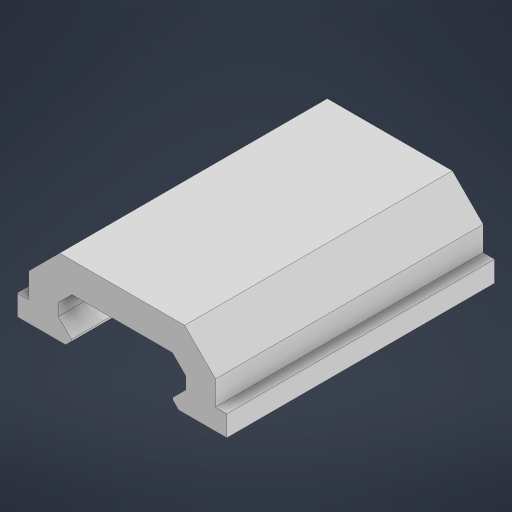
# Autodesk Inventor part: Rail clamp
Saved by Autodesk Inventor 2023 (Build 270158000, 158)
## iProperties
Created: 2023-10-16
Part Number: Rail clamp
Material: Generic
Document SubType Name: Modeling
Designer: nick_
Density: 1 g/cm^3
Appearance: Default
Author: nick_
Autodesk Inventor part; units mm, degrees
ref_plane "YZ Plane" through (0, 0, 0) normal (1, 0, 0) x (0, 1, 0)
ref_plane "XZ Plane" through (0, 0, 0) normal (0, 1, 0) x (-1, 0, 0)
ref_plane "XY Plane" through (0, 0, 0) normal (0, 0, 1) x (1, 0, 0)
sketch "Sketch1" plane through (0, 0, 0) normal (0, 0, 1) x (1, 0, 0)
  line L0 (6.25, -6.1609) -> (-18.75, -6.1609) construction
  line L1 (6.25, -3.1609) -> (6.25, -6.1609) construction
  line L2 (2.1447, -3.1609) -> (6.25, -3.1609) construction
  line L3 (2.1447, -0.2145) -> (2.1447, -3.1609) construction
  line L4 (4.3545, 1.9953) -> (2.1447, -0.2145) construction
  line L5 (4.3545, 3.9511) -> (4.3545, 1.9953) construction
  line L6 (2.1447, 6.1609) -> (4.3545, 3.9511) construction
  line L7 (2.1447, 6.1609) -> (-14.6447, 6.1609) construction
  line L8 (-14.6447, 6.1609) -> (-16.8545, 3.9511) construction
  line L9 (-16.8545, 3.9511) -> (-16.8545, 1.9953) construction
  line L10 (-16.8545, 1.9953) -> (-14.6447, -0.2145) construction
  line L11 (-14.6447, -0.2145) -> (-14.6447, -3.1609) construction
  line L12 (-14.6447, -3.1609) -> (-18.75, -3.1609) construction
  line L13 (-18.75, -3.1609) -> (-18.75, -6.1609) construction
  line L14 (2.2447, -3.0609) -> (6.35, -3.0609)
  line L15 (6.35, -3.0609) -> (6.35, -6.2609)
  line L16 (6.35, -6.2609) -> (-18.85, -6.2609)
  line L17 (-18.85, -6.2609) -> (-18.85, -3.0609)
  line L18 (-18.85, -3.0609) -> (-14.7447, -3.0609)
  line L19 (-14.7447, -3.0609) -> (-14.7447, -0.2559)
  line L20 (-14.7447, -0.2559) -> (-16.9545, 1.9539)
  line L21 (-16.9545, 1.9539) -> (-16.9545, 3.9925)
  line L22 (-16.9545, 3.9925) -> (-14.6861, 6.2609)
  line L23 (-14.6861, 6.2609) -> (2.1861, 6.2609)
  line L24 (2.1861, 6.2609) -> (4.4545, 3.9925)
  line L25 (4.4545, 3.9925) -> (4.4545, 1.9539)
  line L26 (4.4545, 1.9539) -> (2.2447, -0.2559)
  line L27 (2.2447, -0.2559) -> (2.2447, -3.0609)
  line L28 (11.35, 1.9391) -> (9.4545, 1.9391)
  line L29 (9.4545, 1.9391) -> (9.4545, 6.0636)
  line L30 (9.4545, 6.0636) -> (4.2572, 11.2609)
  line L31 (4.2572, 11.2609) -> (-16.7572, 11.2609)
  line L32 (-16.7572, 11.2609) -> (-21.9545, 6.0636)
  line L33 (-21.9545, 6.0636) -> (-21.9545, 1.9391)
  line L34 (-21.9545, 1.9391) -> (-23.85, 1.9391)
  line L35 (-23.85, 1.9391) -> (-23.85, -1.5609)
  line L36 (11.35, -1.5609) -> (11.35, 1.9391)
  line L37 (2.2447, -1.5609) -> (11.35, -1.5609)
  line L38 (-14.7447, -1.5609) -> (-23.85, -1.5609)
  point P0 (0, 0)
  point P1 (6.7974, -1.5609)
  point P2 (-19.2974, -1.5609)
  dimension "d0" = 0.1
  dimension "d1" = 5
  dimension "d2" = 1.5
  dimension "d3" = 5
  dimension "d5" = 5
  constraints: 50 end point, 2 midpoint, 2 perpendicular, 2 point on line, 1 horizontal alignment, 19 other
  measures "d0" distance between parallel lines of L3 L27
  measures "d1" distance between parallel lines of L36 L15
  measures "d2" distance between parallel lines of L37 L14
  measures "d3" distance between parallel lines of L31 L23
  measures "d5" distance between parallel lines of L35 L17
extrude "Extrusion1" add sketch "Sketch1" against normal blind 45 contours L27 L26 L25 L24 L23 L22 L21 L20 L19 L38 L35 L34 L33 L32 L31 L30 L29 L28 L36 L37
chamfer "Chamfer1" distance 1 angle 45 2 edges at (-14.7447, -1.5609, -22.5) (2.2447, -1.5609, -22.5)
equation "\"d5\" = d1"
body "Solid1"
